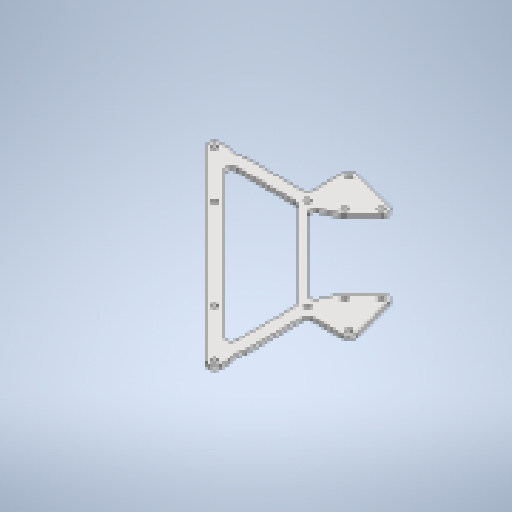
# Autodesk Inventor part: piti_mata
Saved by Autodesk Inventor 2025.1 (Build 291241000, 241)
## iProperties
Created: 2024-08-31
Part Number: piti_mata
Material: 一般
Document SubType Name: Modeling
Designer: right
Density: 1 g/cm^3
Appearance: 既定
Author: right
Autodesk Inventor part; units mm, degrees
ref_plane "YZ Plane" through (0, 0, 0) normal (1, 0, 0) x (0, 1, 0)
ref_plane "XZ Plane" through (0, 0, 0) normal (0, 1, 0) x (-1, 0, 0)
sketch "スケッチ1" plane through (0, 0, 0) normal (0, 1, 0) x (-1, 0, 0)
  line L0 (18, 8) -> (-18, 8) construction
  line L1 (-18, 8) -> (-18, -8) construction
  line L2 (-18, -8) -> (18, -8) construction
  line L3 (18, -8) -> (18, 8) construction
  line L4 (18, 8) -> (-18, -8) construction
  line L5 (-18, 8) -> (18, -8) construction
  circle A0 centre (18, -8) radius 1.1
  circle A1 centre (-18, -8) radius 1.1
  circle A2 centre (-18, 8) radius 1.1
  circle A3 centre (18, -8) radius 2.5
  circle A4 centre (-18, -8) radius 2.5
  circle A5 centre (-18, 8) radius 2.5
  line L6 (18, -10.5) -> (-18, -10.5)
  line L7 (-15.5, 8) -> (-15.5, -8)
  line L8 (-18, -5.5) -> (18, -5.5)
  line L9 (-20.5, -8) -> (-20.5, 8)
  line L10 (-20.5, 0) -> (18, 0) construction
  circle A6 centre (18, 8) radius 1.1
  circle A7 centre (18, 8) radius 2.5
  line L11 (18, 10.5) -> (-18, 10.5)
  line L12 (-18, 5.5) -> (18, 5.5)
  point P0 (0, 0)
  point P1 (-17.0032, -10.2927)
  point P2 (-17.0032, 10.2927)
  point P3 (-15.5, -5.5)
  point P4 (18.123, -10.497)
  point P5 (-15.5, 5.5)
  dimension "d0" = 36
  dimension "d2" = 2.2
  dimension "d3" = 2.2
  dimension "d5" = 5
  dimension "d17" = 16
  constraints: 26 end point, 11 point on circle, 8 centre point, 6 coincident, 5 symmetric about line, 5 tangent, 4 midpoint, 3 equal radius, 2 parallel, 2 perpendicular, 2 point on line, 1 horizontal, 2 other
  measures "d0" distance of L1.end L2.end
  measures "d2" diameter of A0
  measures "d3" diameter of A1
  measures "d5" diameter of A3
  measures "d17" distance of L0.end L1.end
extrude "押し出し1" add sketch "スケッチ1" along normal blind 1.5 contours L8 A4 L9 A5 L12 L7 | L7 A4 L8 | A4 | L12 A5 L7 | L7 A5 L11 A7 L12 | A5 | A7
fillet "フィレット1" radius 2 1 edges at (15.5, 0.75, 5.5)
sketch "スケッチ2" plane through (0, 1.5, 0) normal (0, 1, 0) x (1, 0, 0)
  line L0 (39.5, 8) -> (23.5, -8) construction
  line L1 (20.5, -8) -> (20.5, 8) projected
  circle A0 centre (35.0355, 3.5355) radius 1.1
  circle A1 centre (27.9645, -3.5355) radius 1.1
  line L2 (31.5, 0) -> (34.6629, -3.1629) construction
  circle A2 centre (27.9645, -3.5355) radius 2.5
  circle A3 centre (35.0355, 3.5355) radius 2.5
  line L3 (15.5, 8) -> (15.5, -3.5) projected
  arc A4 (18, -10.5) -> (20.5, -8) centre (18, -8) ccw projected
  line L4 (20.5, -8) -> (20.5, 8) projected
  arc A5 (20.5, 8) -> (15.5, 8) centre (18, 8) ccw projected
  circle A6 centre (18, 8) radius 1.1 projected
  circle A7 centre (18, -8) radius 1.1 projected
  line L5 (18.6338, 10.4183) -> (35.6693, 5.9539)
  line L6 (19.0222, -10.2815) -> (28.9867, -5.817)
  line L7 (36.8033, 1.7678) -> (29.7322, -5.3033)
  line L8 (13.5, -5.5) -> (-18, -5.5) projected
  arc A8 (-18, -5.5) -> (-18, -10.5) centre (-18, -8) ccw projected
  line L9 (-18, -10.5) -> (18, -10.5) projected
  arc A9 (13.5, -5.5) -> (15.5, -3.5) centre (13.5, -3.5) ccw projected
  point P0 (0, 0)
  dimension "d18" = 45
  dimension "d19" = 3
  dimension "d20" = 2.2
  dimension "d21" = 2.2
  dimension "d22" = 5
  dimension "d23" = 5
  dimension "d24" = 5
  dimension "d25" = 5
  constraints: 10 end point, 6 point on circle, 6 tangent, 4 centre point, 2 coincident, 2 horizontal alignment, 2 point on line, 1 midpoint, 1 perpendicular
  measures "d18" angle of L1 L0
  measures "d19" distance of L1.start L0.end
  measures "d20" diameter of A0
  measures "d21" diameter of A1
  measures "d22" distance from line of L2 A0.centre
  measures "d23" distance from line of L2 A1.centre
  measures "d24" diameter of A2
  measures "d25" diameter of A3
extrude "押し出し2" add sketch "スケッチ2" against normal up to surface (1.5 mm away) contours L1 A5 L5 A3 L7 A2 L6 A4 | A2 | A3
ref_plane "作業平面1" through (31.0675, 0, 31.152) normal (0, 1, 0) x (0, 0, 1)
sketch "スケッチ3" plane through (0, 1.5, 0) normal (0, 1, 0) x (1, 0, 0)
  line L0 (36.8033, 5.3033) -> (66.8553, -24.7487) projected
  line L1 (52.1378, -80.9663) -> (-19.4142, -9.4142) projected
  line L2 (51.8293, -9.7227) -> (16.3618, -45.1902) construction
  circle A0 centre (35.0355, 3.5355) radius 1.1 projected
  circle A1 centre (27.9645, -3.5355) radius 1.1 projected
  arc A2 (18, -10.5) -> (19.0222, -10.2815) centre (18, -8) ccw projected
  line L3 (19.0222, -10.2815) -> (28.9867, -5.817) projected
  arc A3 (28.9867, -5.817) -> (29.7322, -5.3033) centre (27.9645, -3.5355) ccw projected
  line L4 (29.7322, -5.3033) -> (36.8033, 1.7678) projected
  arc A4 (36.8033, 1.7678) -> (35.6693, 5.9539) centre (35.0355, 3.5355) ccw projected
  line L5 (35.6693, 5.9539) -> (18.6338, 10.4183) projected
  arc A5 (18.6338, 10.4183) -> (15.5, 8) centre (18, 8) ccw projected
  line L6 (15.5, 8) -> (15.5, -3.5) projected
  arc A6 (13.5, -5.5) -> (15.5, -3.5) centre (13.5, -3.5) ccw projected
  line L7 (13.5, -5.5) -> (-18, -5.5) projected
  arc A7 (-18, -5.5) -> (-18, -10.5) centre (-18, -8) ccw projected
  line L8 (-18, -10.5) -> (18, -10.5) projected
  circle A8 centre (18, -8) radius 1.1 projected
  circle A9 centre (-18, -8) radius 1.1 projected
  circle A10 centre (18, 8) radius 1.1 projected
  line L9 (66.8553, -24.7487) -> (36.8033, 5.3033)
  line L10 (-19.4142, -9.4142) -> (52.1378, -80.9663)
  circle A11 centre (65.0876, -26.5165) radius 1.1
  circle A12 centre (58.0165, -33.5876) radius 1.1
  arc A13 (51.2706, -42.5298) -> (51.052, -43.552) centre (53.552, -43.552) ccw
  line L11 (51.2706, -42.5298) -> (55.735, -32.5654)
  arc A14 (56.2487, -31.8198) -> (55.735, -32.5654) centre (58.0165, -33.5876) ccw
  line L12 (56.2487, -31.8198) -> (63.3198, -24.7487)
  arc A15 (67.5059, -25.8827) -> (63.3198, -24.7487) centre (65.0876, -26.5165) ccw
  line L13 (67.5059, -25.8827) -> (71.9704, -42.9183)
  arc A16 (69.552, -46.052) -> (71.9704, -42.9183) centre (69.552, -43.552) ccw
  line L14 (69.552, -46.052) -> (58.052, -46.052)
  arc A17 (58.052, -46.052) -> (56.052, -48.052) centre (58.052, -48.052) ccw
  line L15 (56.052, -48.052) -> (56.052, -79.552)
  arc A18 (51.052, -79.552) -> (56.052, -79.552) centre (53.552, -79.552) ccw
  line L16 (51.052, -79.552) -> (51.052, -43.552)
  circle A19 centre (53.552, -43.552) radius 1.1
  circle A20 centre (53.552, -79.552) radius 1.1
  circle A21 centre (69.552, -43.552) radius 1.1
  point P0 (0, 0)
  point P1 (61.552, -61.552)
  constraints: 28 symmetric about line, 18 end point, 12 point on circle, 11 centre point, 2 midpoint, 11 other
extrude "押し出し3" add sketch "スケッチ3" against normal up to surface (1.5 mm away) contours A15 L13 A16 L14 A17 L15 A18 L16 A13 L11 A14 L12
sketch "スケッチ4" plane through (0, 1.5, 0) normal (0, 1, 0) x (1, 0, 0)
  arc A0 (51.052, -79.552) -> (56.052, -79.552) centre (53.552, -79.552) ccw projected
  line L0 (51.7843, -81.3198) -> (-19.7678, -9.7678)
  arc A1 (-18, -5.5) -> (-18, -10.5) centre (-18, -8) ccw projected
  arc A2 (-18, -5.5) -> (-18, -10.5) centre (-18, -8) ccw projected
  arc A3 (51.052, -79.552) -> (56.052, -79.552) centre (53.552, -79.552) ccw projected
  circle A4 centre (53.552, -79.552) radius 2.5
  line L1 (55.3198, -77.7843) -> (-16.9645, -5.5)
  line L2 (51.052, -43.552) -> (51.052, -79.552) projected
  line L3 (-18, -10.5) -> (18, -10.5) projected
  line L4 (13.5, -5.5) -> (-18, -5.5) projected
  point P0 (0, 0)
  point P1 (-11.9645, -10.5)
  point P2 (51.052, -73.5165)
  constraints: 4 end point, 2 point on circle, 2 tangent, 1 coincident, 1 parallel, 1 point on line, 5 other
extrude "押し出し5" add sketch "スケッチ4" against normal up to surface (1.5 mm away) contours A0 L0 A1 L3 L1 L2
fillet "フィレット2" radius 2 2 edges at (51.052, 0.75, 73.5165) (-11.9645, 0.75, 10.5)
sketch "スケッチ5" plane through (0, 1.5, 0) normal (0, 1, 0) x (1, 0, 0)
  circle A0 centre (-11.5, 0) radius 6.2325 projected
  circle A1 centre (61.552, -73.052) radius 6.2325 projected
  point P0 (0, 0)
extrude "押し出し6" cut sketch "スケッチ5" against normal through all
sketch "スケッチ6" plane through (0, 1.5, 0) normal (0, 1, 0) x (1, 0, 0)
  line L0 (-7.136, -10.5) -> (18, -10.5) projected
  line L1 (16.3198, -10.5) -> (51.052, -45.2322)
  line L2 (51.052, -68.6881) -> (51.052, -43.552) projected
  line L3 (51.2706, -42.5298) -> (55.735, -32.5654) projected
  line L4 (51.6795, -41.6171) -> (19.935, -9.8725)
  line L5 (28.9867, -5.817) -> (19.0222, -10.2815) projected
  line L6 (47.6378, -70.1023) -> (-8.5503, -13.9142) projected
  arc A0 (18, -10.5) -> (19.0222, -10.2815) centre (18, -8) ccw projected
  arc A1 (51.2706, -42.5298) -> (51.052, -43.552) centre (53.552, -43.552) ccw projected
  point P0 (0, 0)
  dimension "d37" = 3
  dimension "d38" = 20
  constraints: 4 end point, 4 point on line, 2 parallel
  measures "d37" distance between parallel lines of L1 L4
  measures "d38" distance between parallel lines of L6 L1
extrude "押し出し7" add sketch "スケッチ6" against normal up to surface (1.5 mm away)
fillet "フィレット3" radius 2 4 edges at (16.3198, 0.75, 10.5) (19.935, 0.75, 9.8725) (51.052, 0.75, 45.2322) (51.6795, 0.75, 41.6171)
sketch "スケッチ7" plane through (0, 1.5, 0) normal (0, 1, 0) x (1, 0, 0)
  arc A0 (-7.136, -10.5) -> (-8.5503, -13.9142) centre (-7.136, -12.5) ccw construction
  line L0 (-8.5503, -13.9142) -> (-12.0858, -17.4497) construction
  line L1 (-19.7678, -9.7678) -> (51.7843, -81.3198) construction
  line L2 (-10.318, -15.682) -> (45.8701, -71.8701) construction
  arc A1 (47.6378, -70.1023) -> (51.052, -68.6881) centre (49.052, -68.6881) ccw construction
  line L3 (47.6378, -70.1023) -> (44.1023, -73.6378) construction
  circle A2 centre (0.2886, -26.2886) radius 1.1
  line L4 (47.6378, -70.1023) -> (-8.5503, -13.9142) projected
  line L5 (17.776, -43.776) -> (16.0083, -45.5438) construction
  circle A3 centre (35.2635, -61.2635) radius 1.1
  point P0 (0, 0)
  dimension "d42" = 2.2
  dimension "d43" = 15
  constraints: 8 end point, 4 midpoint, 3 point on line, 2 centre point, 2 perpendicular, 1 parallel, 1 symmetric about line, 1 other
  measures "d42" diameter of A2
  measures "d43" distance from line of L0 A2.centre
extrude "押し出し8" cut sketch "スケッチ7" against normal through all
equation "\"d23\" = d22"
equation "\"d24\" = d25"
equation "\"d26\" = d22"
